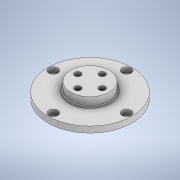
# Autodesk Inventor part: Output2
Saved by Autodesk Inventor 2021 (Build 250183000, 183)
## iProperties
Created: 2022-08-14
Part Number: Output2
Material: Ogólny
Document SubType Name: Modeling
Designer: MicnedSQ
Density: 1 g/cm^3
Appearance: Domyślna
Author: MicnedSQ
## iProperties of the stored document _Drukowanie 3D.ipt
Created: 2022-08-14
Part Number: _Drukowanie 3D
Material: Ogólny
Document SubType Name: Modeling
Designer: MicnedSQ
Density: 1 g/cm^3
Appearance: Domyślna
Author: MicnedSQ
Autodesk Inventor part; units mm, degrees
ref_plane "YZ Plane" through (0, 0, 0) normal (1, 0, 0) x (0, 1, 0)
ref_plane "XZ Plane" through (0, 0, 0) normal (0, 1, 0) x (-1, 0, 0)
ref_plane "XY Plane" through (0, 0, 0) normal (0, 0, 1) x (1, 0, 0)
sketch "Szkic1" plane through (0, 0, 0) normal (0, 1, 0) x (-1, 0, 0)
  circle A0 centre (0, 0) radius 27.5
  dimension "d0" = 55
  constraints: 1 centre point, 1 coincident
  measures "d0" diameter of A0
extrude "Wyciągnięcie proste1" add sketch "Szkic1" along normal blind 4
sketch "Szkic2" plane through (0, 4, 0) normal (0, 1, 0) x (1, 0, 0)
  circle A0 centre (-24, 0) radius 1.55
  circle A1 centre (0, -24) radius 1.55
  circle A2 centre (24, 0) radius 1.55
  circle A3 centre (0, 24) radius 1.55
  point P0 (0, 0)
  dimension "d3" = 3.1
  dimension "d4" = 24
  dimension "d7" = 360
  constraints: 4 centre point, 9 other
  measures "d3" diameter of A0
  measures "d4" distance of point (0, 0) A0.centre
extrude "Wyciągnięcie proste2" cut sketch "Szkic2" against normal up to surface (4 mm away)
sketch "Szkic3" plane through (0, 4, 0) normal (0, 1, 0) x (1, 0, 0)
  circle A0 centre (0, 0) radius 12.5
  dimension "d11" = 25
  constraints: 1 centre point, 1 coincident
  measures "d11" diameter of A0
extrude "Wyciągnięcie proste3" add sketch "Szkic3" along normal blind 6
sketch "Szkic4" plane through (0, 10, 0) normal (0, 1, 0) x (1, 0, 0)
  circle A0 centre (-8, 0) radius 2.05
  circle A1 centre (0, -8) radius 2.05
  circle A2 centre (8, 0) radius 2.05
  circle A3 centre (0, 8) radius 2.05
  point P0 (0, 0)
  dimension "d14" = 4.1
  dimension "d17" = 360
  dimension "d19" = 8
  constraints: 4 centre point, 9 other
  measures "d14" diameter of A0
  measures "d19" distance of point (0, 0) A0.centre
extrude "Wyciągnięcie proste4" cut sketch "Szkic4" against normal blind 8
sketch "Szkic5" plane through (0, 4, 0) normal (0, 1, 0) x (1, 0, 0)
  circle A0 centre (-24, 0) radius 1.55 projected
  circle A1 centre (-24, 0) radius 3
  circle A2 centre (0, -24) radius 3
  circle A3 centre (24, 0) radius 3
  circle A4 centre (0, 24) radius 3
  point P0 (0, 0)
  dimension "d22" = 6
  dimension "d27" = 360
  constraints: 4 centre point, 1 coincident, 9 other
  measures "d22" diameter of A1
extrude "Wyciągnięcie proste5" cut sketch "Szkic5" against normal blind 3.2
sketch "Szkic6" plane through (0, 4, 0) normal (0, 1, 0) x (1, 0, 0)
  circle A0 centre (0, 0) radius 13.5
  dimension "d29" = 27
  constraints: 1 centre point, 1 coincident
  measures "d29" diameter of A0
extrude "Wyciągnięcie proste6" add sketch "Szkic6" along normal blind 1
